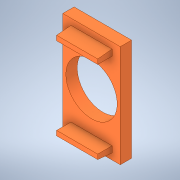
# Autodesk Inventor part: 20_Cube_insert_Sample_holder
Saved by Autodesk Inventor 2022 (Build 260153000, 153)
## iProperties
Created: 2019-08-07
Part Number: 20_Cube_insert_Sample_holder
Material: Generic
Document SubType Name: Modeling
Designer: marsikovabarbora
Density: 1 g/cm^3
Appearance: Default
Author: marsikovabarbora
Autodesk Inventor part; units mm, degrees
ref_plane "XZ Plane" through (0, 0, 0) normal (0, 1, 0) x (-1, 0, 0)
ref_plane "XY Plane" through (0, 0, 0) normal (0, 0, 1) x (1, 0, 0)
sketch "Sketch1" plane through (0, 0, 0) normal (0, 0, 1) x (1, 0, 0)
  line L0 (0, -35.8) -> (0, 40.5) construction
  line L1 (0, 0) -> (11.1575, 11.1575) construction
  line L2 (0, 0) -> (15.7791, 0) construction
  line L3 (0, 24.9) -> (14, 24.9)
  line L4 (14, 24.9) -> (14, 21.2415)
  line L5 (2.8009, -24.9) -> (14, -24.9)
  line L6 (14, -24.9) -> (14, -21.2415)
  line L7 (0, 24.9) -> (-14, 24.9)
  line L8 (-14, 24.9) -> (-14, 21.2415)
  line L9 (2.8009, -24.9) -> (-14, -24.9)
  line L10 (-14, -24.9) -> (-14, -21.2415)
  circle A0 centre (0, 0) radius 12.5
  line L11 (14, 24.9) -> (14, -21.2415)
  line L12 (-14, 21.2415) -> (-14, -21.2415)
  dimension "d0" = 45
  dimension "d5" = 25
  dimension "d19" = 28
  constraints: 24 end point, 4 symmetric about line, 2 horizontal, 1 centre point, 1 coincident, 1 equal length, 1 perpendicular, 1 point on line, 1 vertical
  measures "d0" angle of L2 L1
  measures "d5" diameter of A0
  measures "d19" distance between parallel lines of L12 L11
extrude "Extrusion1" add sketch "Sketch1" along normal blind 5.5
sketch "Sketch2" plane through (0, 0, 5.5) normal (0, 0, 1) x (1, 0, 0)
  circle A0 centre (0, 0) radius 12.5 projected
  line L0 (14, 24.9) -> (-14, 24.9) projected
  line L1 (-14, 24.9) -> (-14, -24.9) projected
  line L2 (-14, -24.9) -> (14, -24.9) projected
  line L3 (14, -24.9) -> (14, 24.9) projected
  line L4 (-37.0494, 0) -> (27.1749, 0) construction
  line L5 (0, -35.8) -> (0, 40.5) construction
  line L6 (-10, 21.9) -> (10, 21.9)
  line L7 (10, 21.9) -> (10, 18.9)
  line L8 (10, 18.9) -> (-10, 18.9)
  line L9 (-10, 18.9) -> (-10, 21.9)
  line L10 (-10, -21.9) -> (10, -21.9)
  line L11 (10, -21.9) -> (10, -18.9)
  line L12 (10, -18.9) -> (-10, -18.9)
  line L13 (-10, -18.9) -> (-10, -21.9)
  dimension "d8" = 20
  dimension "d9" = 3
  dimension "d10" = 3
  dimension "d20" = 18.9
  dimension "d21" = 18.9
  constraints: 16 end point, 4 symmetric about line, 2 parallel, 1 horizontal, 1 perpendicular, 1 other
  measures "d8" distance of L6.start L6.end
  measures "d9" distance of L6.end L7.end
  measures "d10" distance between parallel lines of L6 L0
  measures "d20" distance from line of L8 point (0, 0)
  measures "d21" distance from line of L12 point (0, 0)
extrude "Extrusion2" add sketch "Sketch2" along normal blind 7 contours L6 L7 L8 L9 | L13 L12 L11 L10
chamfer "Fase1" distance 0.7 distance2 7 1 edges at (0, 21.9, 12.5) measured on face at (-3.3333, 19.9, 12.5)
chamfer "Fase2" distance 0.7 distance2 7 1 edges at (0, -21.9, 12.5) measured on face at (-3.3333, -19.9, 12.5)
sketch "Skizze4" plane through (0, 0, 0) normal (0, 0, -1) x (-1, 0, 0)
  line L0 (10, -18.9) -> (-10, -18.9) projected
  line L1 (-10, 18.9) -> (10, 18.9) projected
  line L2 (10, -18.9) -> (-10, -18.9)
  line L3 (-10, -18.9) -> (-10, 18.9) construction
  line L4 (-10, 18.9) -> (10, 18.9)
  line L5 (10, 18.9) -> (10, -18.9)
  line L6 (-10, -21.9) -> (10, -21.9) projected
  line L7 (-10, -18.9) -> (10, -18.9)
  line L8 (10, -18.9) -> (10, -21.9)
  line L9 (10, -21.9) -> (-10, -21.9)
  line L10 (-10, -21.9) -> (-10, -18.9)
  point P0 (0, 0)
  point P1 (10, -20.4)
  point P2 (0, 0)
  point P3 (-10, -17)
  dimension "d22" = 18.9
  dimension "d23" = 20
  dimension "d24" = 3
  dimension "d33" = 17
  constraints: 16 end point, 4 equal length, 2 horizontal, 2 perpendicular, 1 coincident, 1 midpoint, 1 point on line
  measures "d22" distance from line of L0 point (0, 0)
  measures "d24" distance between parallel lines of L6 L0
  measures "d33" vertical distance of point (-10, -17) point (0, 0)
ref_plane "Arbeitsebene2" through (10, -17, 0) normal (1, 0, 0) x (0, 1, 0)
sketch "Skizze5" plane through (10, -20.4, 0) normal (0, 0, -1) x (0, 1, 0)
  line L0 (50, 0.0005) -> (0, 0.0005)
  point P0 (20.4, -10)
  point P1 (25, 0)
  point P2 (40, 8)
  point P3 (6.6949, -37.8745)
  point P4 (0, 0.0005)
  constraints: 3 other
sketch "Skizze6" plane through (10, -17, 0) normal (1, 0, 0) x (0, 1, 0)
  line L0 (50, -0.1341) -> (0, -0.1341)
  line L1 (-5, 0.0159) -> (-5, 5.0159)
  line L2 (0, -0.1341) -> (0, 5.1659)
  line L3 (0, 1.0159) -> (2.1846, 1.0159)
  line L4 (-2.3, -1.5874) -> (-2.3, 1.1997)
  line L5 (0, -1.5874) -> (0, -0.1341)
  arc A0 (-2.3, 3.8322) -> (-0.8789, 0.0159) centre (0, 2.5159) ccw
  arc A1 (0, -0.1341) -> (0, 5.1659) centre (0, 2.5159) ccw
  line L6 (2.1846, 1.0159) -> (3.3346, -0.1341)
  line L7 (3.3346, -0.1341) -> (0, -0.1341)
  line L8 (0, 2.5159) -> (1.8859, 2.5159)
  line L9 (2.1846, 4.0159) -> (3.3346, 5.1659)
  line L10 (3.3346, 5.1659) -> (0, 5.1659)
  point P0 (17, 0)
  point P1 (25, 0)
  point P2 (40, 8)
  point P3 (6.6949, -37.8745)
  point P4 (0, -0.1341)
  dimension "d34" = 2.65
  dimension "d35" = 5
  dimension "d36" = 2.3
  dimension "d37" = 135
  dimension "d38" = 1.5
  dimension "d39" = 2.65
  constraints: 20 end point, 7 point on circle, 3 horizontal, 2 centre point, 2 point on line, 1 perpendicular, 1 vertical, 3 other
  measures "d35" distance from line of L1 L8.start
  measures "d36" distance between parallel lines of L4 L2
  measures "d37" angle of L7 L6
  measures "d38" distance from line of L8.start L3
  measures "d39" radius of A1
revolve "Umdrehung2" cut sketch "Skizze6" angle 360 about axis through (10, -17, -0.1341) along (0, 0, 1)
mirror "Spiegeln3" about plane through (0, 0, 0) normal (1, 0, 0) of "Umdrehung2"
mirror "Spiegeln4" about plane through (0, 0, 0) normal (0, 1, 0) of "Umdrehung2", "Spiegeln3"
body "Solid1"
